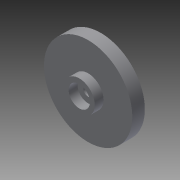
# Autodesk Inventor part: Horn
Saved by Autodesk Inventor 2015 SP1 (Build 190203100, 203)
## iProperties
Created: 2015-03-15
Part Number: Horn
Material: Generic
Document SubType Name: Modeling
Designer: fuji
Density: 1 g/cm^3
Appearance: Default
Author: fuji
Autodesk Inventor part; units mm, degrees
ref_plane "YZ Plane" through (0, 0, 0) normal (1, 0, 0) x (0, 1, 0)
ref_plane "XZ Plane" through (0, 0, 0) normal (0, 1, 0) x (-1, 0, 0)
ref_plane "XY Plane" through (0, 0, 0) normal (0, 0, 1) x (1, 0, 0)
sketch "Sketch1" plane through (0, 0, 0) normal (0, 0, 1) x (1, 0, 0)
  circle A0 centre (0, 0) radius 12.7
  circle A1 centre (0, 0) radius 1.397
  dimension "d0" = 25.4
  dimension "d1" = 2.794
  constraints: 2 centre point, 2 coincident
  measures "d0" diameter of A0
  measures "d1" diameter of A1
extrude "Extrusion1" add sketch "Sketch1" along normal blind 1.5875
sketch "Sketch2" plane through (0, 0, 1.5875) normal (0, 0, 1) x (1, 0, 0)
  circle A0 centre (0, 0) radius 3.048
  circle A1 centre (0, 0) radius 4.445
  dimension "d4" = 6.096
  dimension "d5" = 8.89
  constraints: 2 centre point, 2 coincident
  measures "d4" diameter of A0
  measures "d5" diameter of A1
extrude "Extrusion2" add sketch "Sketch2" along normal blind 2.54
sketch "Sketch3" plane through (0, 0, 0) normal (0, 0, -1) x (-1, 0, 0)
  circle A0 centre (0, 0) radius 12.7
  circle A1 centre (0, 0) radius 5.1432
  dimension "d8" = 25.4
  constraints: 2 centre point, 2 coincident
  measures "d8" diameter of A0
extrude "Extrusion3" add sketch "Sketch3" along normal blind 2.032
equation "\"d0\" = hornD"
equation "\"d1\" = hornS"
equation "\"d2\" = hornT"
equation "\"d4\" = hornID"
equation "\"d5\" = hornOD"
equation "\"d6\" = hornH"
equation "\"d8\" = spoolD"
equation "\"d9\" = inset"
equation "\"spoolD\" = 25.4"
equation "\"hubD\" = 6.35"
equation "\"spoolT\" = 1.5875"
equation "\"hubH\" = 6.35"
equation "\"hornD\" = 25.4"
equation "\"hornT\" = 1.5875"
equation "\"hornS\" = 2.794"
equation "\"hornID\" = 6.096"
equation "\"hornOD\" = 8.89"
equation "\"hornH\" = 2.54"
equation "\"inset\" = 2.032"
equation "\"insetD\" = 5.842"
body "Solid1"
